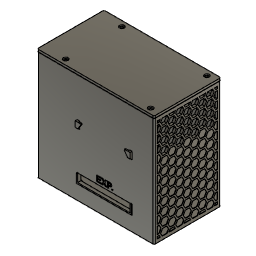
book8088_isa_exp_encloser_typeA (Autodesk Fusion 360 design; units mm, degrees)
Autodesk Fusion 360 part; units mm, degrees
(part 1 of 3)
sketch "스케치1" plane through (0, 0, 0) normal (0, 0, 1) x (1, 0, 0)
  line L0 (0, 75.3) -> (90.25, 75.3)
  line L1 (90.25, 75.3) -> (90.25, 0) construction
  line L2 (90.25, 0) -> (0, 0)
  line L3 (0, 0) -> (0, 75.3) construction
  line L4 (1.75, 0) -> (22.5, 0)
  line L5 (0, 1.75) -> (0, 22.5)
  line L6 (4.35, 70.95) -> (4.35, 4.35) construction
  line L7 (85.9, 70.95) -> (85.9, 4.35) construction
  line L8 (4.35, 70.95) -> (85.9, 70.95) construction
  line L9 (4.35, 4.35) -> (85.9, 4.35) construction
  circle A0 centre (4.35, 70.95) radius 1.55
  circle A1 centre (4.35, 70.95) radius 5
  circle A2 centre (85.9, 70.95) radius 1.55
  circle A3 centre (85.9, 70.95) radius 5
  circle A4 centre (85.9, 4.35) radius 1.55
  circle A5 centre (85.9, 4.35) radius 5
  circle A6 centre (4.35, 4.35) radius 1.55
  circle A7 centre (4.35, 4.35) radius 5
  line L10 (-37, 78.3) -> (105.25, 78.3)
  line L11 (105.25, 78.3) -> (105.25, -3)
  line L12 (105.25, -3) -> (-37, -3)
  line L13 (-37, -3) -> (-37, 78.3)
  line L14 (102.25, 75.3) -> (102.25, 0)
  line L15 (90.25, 75.3) -> (102.25, 75.3)
  line L16 (102.25, 0) -> (90.25, 0)
  line L17 (-34, 75.3) -> (-34, 0)
  line L18 (-34, 75.3) -> (0, 75.3)
  line L19 (-34, 0) -> (0, 0)
  line L20 (-22.25, 75.3) -> (-22.25, 0)
  line L21 (-25.75, 75.3) -> (-25.75, 0)
  line L22 (-22.25, 67.225) -> (-25.75, 67.225)
  line L23 (-25.75, 54.875) -> (-22.25, 54.875)
  line L24 (-25.75, 46.825) -> (-22.25, 46.825)
  line L25 (-25.75, 34.475) -> (-22.25, 34.475)
  line L26 (-25.75, 26.425) -> (-22.25, 26.425)
  line L27 (-22.25, 14.075) -> (-25.75, 14.075)
  line L28 (-22.25, 54.875) -> (-19.75, 54.875)
  line L29 (-19.75, 54.875) -> (-19.75, 67.225)
  line L30 (-19.75, 67.225) -> (-22.25, 67.225)
  line L31 (-22.25, 46.825) -> (-19.75, 46.825)
  line L32 (-19.75, 46.825) -> (-19.75, 34.475)
  line L33 (-19.75, 34.475) -> (-22.25, 34.475)
  line L34 (-22.25, 26.425) -> (-19.75, 26.425)
  line L35 (-19.75, 26.425) -> (-19.75, 14.075)
  line L36 (-19.75, 14.075) -> (-22.25, 14.075)
  circle A8 centre (-27.33, 69.325) radius 1.5
  line L37 (-34, 67.825) -> (-25.75, 67.825) construction
  line L38 (-25.83, 75.3) -> (-25.83, 0) construction
  line L39 (-33.7, 47.425) -> (-26.25, 47.425) construction
  circle A9 centre (-27.33, 48.925) radius 1.5
  circle A10 centre (-27.33, 28.525) radius 1.5
  line L40 (-33.7, 27.025) -> (-26.25, 27.025) construction
  line L41 (2.65, 59.35) -> (87.9, 59.35) construction
  line L42 (87.9, 59.35) -> (87.9, 50.4) construction
  line L43 (87.9, 50.4) -> (2.65, 50.4) construction
  line L44 (2.65, 50.4) -> (2.65, 59.35) construction
  line L45 (87.9, 30) -> (2.65, 30) construction
  line L46 (2.65, 38.95) -> (87.9, 38.95) construction
  line L47 (2.65, 30) -> (2.65, 38.95) construction
  line L48 (87.9, 38.95) -> (87.9, 30) construction
  line L49 (87.9, 9.6) -> (2.65, 9.6) construction
  line L50 (2.65, 18.55) -> (87.9, 18.55) construction
  line L51 (2.65, 9.6) -> (2.65, 18.55) construction
  line L52 (87.9, 18.55) -> (87.9, 9.6) construction
  line L53 (2.65, 54.875) -> (87.9, 54.875) construction
  line L54 (2.65, 34.475) -> (87.9, 34.475) construction
  line L55 (2.65, 14.075) -> (87.9, 14.075) construction
  line L56 (96.25, 59.35) -> (102.25, 59.35)
  line L57 (96.25, 50.4) -> (102.25, 50.4)
  line L58 (96.25, 59.35) -> (96.25, 56.375)
  line L59 (96.25, 56.375) -> (99.75, 56.375)
  line L60 (99.75, 56.375) -> (99.75, 53.375)
  line L61 (99.75, 53.375) -> (96.25, 53.375)
  line L62 (96.25, 53.375) -> (96.25, 50.4)
  line L63 (96.25, 38.95) -> (102.25, 38.95)
  line L64 (96.25, 38.95) -> (96.25, 35.975)
  line L65 (96.25, 35.975) -> (99.75, 35.975)
  line L66 (99.75, 35.975) -> (99.75, 32.975)
  line L67 (99.75, 32.975) -> (96.25, 32.975)
  line L68 (96.25, 32.975) -> (96.25, 30)
  line L69 (96.25, 30) -> (102.25, 30)
  line L70 (96.25, 18.55) -> (102.25, 18.55)
  line L71 (96.25, 18.55) -> (96.25, 15.575)
  line L72 (96.25, 15.575) -> (99.75, 15.575)
  line L73 (99.75, 15.575) -> (99.75, 12.575)
  line L74 (99.75, 12.575) -> (96.25, 12.575)
  line L75 (96.25, 12.575) -> (96.25, 9.6)
  line L76 (96.25, 9.6) -> (102.25, 9.6)
  line L77 (11.625, 0) -> (11.625, -3) construction
  line L78 (78.625, 0) -> (78.625, -3) construction
  line L79 (45.125, 0) -> (45.125, -3) construction
  line L80 (10.25, 78.3) -> (10.25, 75.3) construction
  line L81 (17.95, 78.3) -> (17.95, 75.3) construction
  line L82 (-37, 75.3) -> (-34, 75.3)
  line L83 (-37, 0) -> (-34, 0)
  line L84 (-22.25, 69.225) -> (-17.75, 69.225)
  line L85 (-17.75, 69.225) -> (-17.75, 52.875)
  line L86 (-17.75, 52.875) -> (-22.25, 52.875)
  line L87 (-17.75, 61.05) -> (-19.75, 61.05) construction
  line L88 (-22.25, 48.825) -> (-17.75, 48.825)
  line L89 (-17.75, 48.825) -> (-17.75, 32.475)
  line L90 (-17.75, 40.65) -> (-19.75, 40.65) construction
  line L91 (-17.75, 32.475) -> (-22.25, 32.475)
  line L92 (-22.25, 28.425) -> (-17.75, 28.425)
  line L93 (-17.75, 28.425) -> (-17.75, 12.075)
  line L94 (-17.75, 20.25) -> (-19.75, 20.25) construction
  line L95 (-17.75, 12.075) -> (-22.25, 12.075)
  line L96 (-37, 9.6) -> (-22.25, 9.6)
  line L97 (91.25, 0) -> (91.25, 7)
  line L98 (91.25, 7) -> (98.25, 7)
  line L99 (98.25, 7) -> (98.25, 0)
  circle A11 centre (94.75, 3.5) radius 3.5 construction
  circle A12 centre (94.75, 3.5) radius 1.5
  line L100 (91.25, 75.3) -> (91.25, 68.3)
  line L101 (91.25, 68.3) -> (98.25, 68.3)
  line L102 (98.25, 68.3) -> (98.25, 75.3)
  circle A13 centre (94.75, 71.8) radius 3.5 construction
  circle A14 centre (94.75, 71.8) radius 1.5
  line L103 (-12.25, 7) -> (-12.25, 0)
  line L104 (-12.25, 7) -> (-5.25, 7)
  line L105 (-5.25, 7) -> (-5.25, 0)
  line L106 (-12.25, 75.3) -> (-12.25, 68.3)
  line L107 (-12.25, 68.3) -> (-5.25, 68.3)
  line L108 (-5.25, 68.3) -> (-5.25, 75.3)
  circle A15 centre (-8.75, 71.8) radius 3.5 construction
  circle A16 centre (-8.75, 3.5) radius 3.5 construction
  circle A17 centre (-8.75, 3.5) radius 1.5
  circle A18 centre (-8.75, 71.8) radius 1.5
  dimension "d1" = 90.25
  dimension "d2" = 75.3
  dimension "d3" = 4.35
  dimension "d4" = 4.35
  dimension "d5" = 4.35
  dimension "d6" = 4.35
  dimension "d8" = 81.55
  dimension "d9" = 3.1
  dimension "d10" = 10
  dimension "d11" = 3
  dimension "d12" = 3
  dimension "d13" = 37
  dimension "d14" = 15
  dimension "d15" = 3
  dimension "d16" = 3
  dimension "d17" = 22.25
  dimension "d18" = 3.5
  dimension "d21" = 12.35
  dimension "d24" = 8.05
  dimension "d25" = 8.05
  dimension "d26" = 2.5
  dimension "d27" = 3
  dimension "d28" = 0.6
  dimension "d33" = 0.6
  dimension "d34" = 0.6
  dimension "d36" = 8.95
  dimension "d38" = 85.25
  dimension "d43" = 1.7
  dimension "d44" = 9.6
  dimension "d46" = 3
  dimension "d47" = 6
  dimension "d48" = 3.5
  dimension "d55" = 67
  dimension "d56" = 7.7
  dimension "d57" = 5.9
  dimension "d94" = 2
  dimension "d95" = 2
  dimension "d104" = 3.58
  dimension "d146" = 7
  dimension "d147" = 7
  dimension "d149" = 3
  dimension "d150" = 4
  dimension "d151" = 10
  constraint horizontal L0
  constraint vertical L1
  constraint horizontal L2
  constraint vertical L3
  constraint collinear L2 L4
  constraint collinear L3 L5
  constraint perpendicular L2 L6
  constraint horizontal L8
  constraint horizontal L9
  constraint equal L8 L9
  constraint equal L6 L7
  constraint perpendicular L7 L8
  constraint coincident L6 L8.start
  constraint coincident L8 L6.start
  constraint concentric A0 A1
  constraint equal A0 A2
  constraint equal A0 A6
  constraint equal A0 A4
  constraint equal A1 A3
  constraint equal A1 A7
  constraint equal A1 A5
  constraint coincident L7 L8.end
  constraint coincident L8 L7.start
  constraint coincident L7 L9.end
  constraint coincident L9 L7.end
  constraint coincident L9 L6.end
  constraint coincident L6 L9.start
  constraint concentric A2 A3
  constraint concentric A4 A5
  constraint concentric A6 A7
  constraint coincident L7.end L9.end
  constraint coincident L7.start L8.end
  constraint coincident L6.start L8.start
  constraint coincident L6.end L9.start
  constraint horizontal L10
  constraint perpendicular L10 L11
  constraint perpendicular L11 L12
  constraint perpendicular L10 L13
  constraint coincident L10.start L13.end
  constraint parallel L1 L14
  constraint perpendicular L1 L15
  constraint collinear L0 L15
  constraint coincident L0.end L1.start
  constraint coincident L14.start L15.end
  constraint horizontal L16
  constraint collinear L2 L16
  constraint coincident L1.end L2.start
  constraint coincident L14.end L16.start
  constraint perpendicular L12 L17
  constraint coincident L2.end L3.start
  constraint collinear L0 L18
  constraint collinear L2 L19
  constraint parallel L17 L20
  constraint coincident L18 L20.start
  constraint coincident L19 L20.end
  constraint parallel L20 L21
  constraint coincident L18 L21.start
  constraint coincident L19 L21.end
  constraint coincident L20 L22.start
  constraint coincident L21 L22.end
  constraint perpendicular L21 L22
  constraint coincident L21 L23.start
  constraint coincident L20 L23.end
  constraint perpendicular L20 L23
  constraint coincident L21 L24.start
  constraint coincident L20 L24.end
  constraint perpendicular L20 L24
  constraint coincident L21 L25.start
  constraint coincident L20 L25.end
  constraint perpendicular L20 L25
  constraint coincident L21 L26.start
  constraint coincident L20 L26.end
  constraint perpendicular L20 L26
  constraint coincident L20 L27.start
  constraint coincident L21 L27.end
  constraint perpendicular L21 L27
  constraint perpendicular L20 L28
  constraint perpendicular L23 L29
  constraint perpendicular L24 L32
  constraint perpendicular L26 L35
  constraint collinear L26 L34
  constraint collinear L27 L36
  constraint collinear L25 L33
  constraint collinear L24 L31
  constraint collinear L22 L30
  constraint equal L30 L31
  constraint equal L30 L34
  constraint horizontal L37
  constraint tangent A8 L37
  constraint coincident L21 L37.end
  constraint coincident L17 L37.start
  constraint vertical L38
  constraint tangent A8 L38
  constraint coincident L18 L38.start
  constraint coincident L19 L38.end
  constraint horizontal L39
  constraint tangent L39 A9
  constraint horizontal L40
  constraint tangent A10 L40
  constraint equal A8 A9
  constraint equal A8 A10
  constraint horizontal L41
  constraint vertical L42
  constraint horizontal L43
  constraint vertical L44
  constraint equal L29 L32
  constraint equal L29 L35
  constraint horizontal L46
  constraint vertical L48
  constraint horizontal L45
  constraint vertical L47
  constraint horizontal L50
  constraint vertical L52
  constraint horizontal L49
  constraint vertical L51
  constraint equal L41 L45
  constraint equal L41 L50
  constraint equal L42 L48
  constraint equal L42 L52
  constraint collinear L42 L48
  constraint collinear L42 L52
  constraint parallel L0 L53
  constraint symmetric L41 L43 L53
  constraint coincident L44 L53.start
  constraint coincident L42 L53.end
  constraint symmetric L45 L46 L54
  constraint symmetric L49 L50 L55
  constraint coincident L47 L54.start
  constraint coincident L48 L54.end
  constraint coincident L52 L55.end
  constraint coincident L51 L55.start
  constraint collinear L36 L55
  constraint collinear L33 L54
  constraint collinear L28 L53
  constraint perpendicular L1 L56
  constraint perpendicular L1 L57
  constraint equal L56 L57
  constraint collinear L41 L56
  constraint collinear L43 L57
  constraint coincident L14 L56.end
  constraint coincident L14 L57.end
  constraint perpendicular L56 L58
  constraint perpendicular L1 L59
  constraint perpendicular L59 L60
  constraint perpendicular L1 L61
  constraint perpendicular L57 L62
  constraint symmetric L53 L59 L61
  constraint equal L63 L69
  constraint perpendicular L63 L64
  constraint perpendicular L65 L66
  constraint perpendicular L68 L69
  constraint equal L70 L76
  constraint perpendicular L70 L71
  constraint perpendicular L72 L73
  constraint perpendicular L75 L76
  constraint coincident L14 L63.end
  constraint coincident L14 L69.end
  constraint coincident L14 L70.end
  constraint coincident L14 L76.end
  constraint collinear L46 L63
  constraint collinear L45 L69
  constraint collinear L50 L70
  constraint collinear L49 L76
  constraint symmetric L55 L72 L74
  constraint symmetric L54 L65 L67
  constraint perpendicular L66 L67
  constraint perpendicular L73 L74
  constraint equal L56 L63
  constraint equal L59 L65
  constraint equal L60 L66
  constraint equal L56 L70
  constraint equal L59 L72
  constraint equal L60 L73
  constraint coincident L2 L77.start
  constraint coincident L12 L77.end
  constraint perpendicular L12 L77
  constraint coincident L2 L78.start
  constraint coincident L12 L78.end
  constraint perpendicular L12 L78
  constraint coincident L2 L79.start
  constraint coincident L12 L79.end
  constraint perpendicular L12 L79
  constraint symmetric L77 L78 L79
  constraint symmetric L6 L7 L79
  constraint coincident L10 L80.start
  constraint coincident L0 L80.end
  constraint perpendicular L0 L80
  constraint coincident L10 L81.start
  constraint coincident L0 L81.end
  constraint perpendicular L0 L81
  constraint perpendicular L13 L82
  constraint collinear L18 L82
  constraint coincident L17.start L18.start
  constraint coincident L13 L82.start
  constraint horizontal L83
  constraint collinear L19 L83
  constraint coincident L17.end L19.start
  constraint coincident L13 L83.start
  constraint tangent L38 A9
  constraint tangent L38 A10
  constraint coincident L20 L84.start
  constraint perpendicular L20 L84
  constraint perpendicular L10 L85
  constraint coincident L20 L86.end
  constraint perpendicular L20 L86
  constraint coincident L85 L87.start
  constraint coincident L29 L87.end
  constraint perpendicular L29 L87
  constraint symmetric L28 L30 L87
  constraint symmetric L84 L86 L87
  constraint coincident L90.start L89
  constraint symmetric L88 L90 L91
  constraint coincident L94.start L93
  constraint symmetric L92 L94 L95
  constraint coincident L20 L88.start
  constraint coincident L32 L90.end
  constraint coincident L20 L91.end
  constraint coincident L20 L92.start
  constraint coincident L35 L94.end
  constraint coincident L20 L95.end
  constraint symmetric L34 L36 L94
  constraint symmetric L31 L33 L90
  constraint perpendicular L93 L95
  constraint perpendicular L92 L93
  constraint perpendicular L89 L91
  constraint perpendicular L88 L89
  constraint equal L87 L90
  constraint equal L87 L94
  constraint equal L85 L89
  constraint equal L85 L93
  constraint perpendicular L17 L96
  constraint collinear L49 L96
  constraint coincident L20 L96.end
  constraint coincident L13 L96.start
  constraint perpendicular L9 L97
  constraint perpendicular L97 L98
  constraint perpendicular L98 L99
  constraint coincident L2 L99.end
  constraint coincident L2 L97.start
  constraint tangent L98 A11
  constraint tangent L99 A11
  constraint tangent L97 A11
  constraint concentric A11 A12
  constraint perpendicular L8 L100
  constraint perpendicular L100 L101
  constraint perpendicular L8 L102
  constraint coincident L0 L100.start
  constraint coincident L0 L102.end
  constraint equal L98 L101
  constraint equal L99 L102
  constraint tangent L102 A13
  constraint tangent L101 A13
  constraint tangent L100 A13
  constraint concentric A13 A14
  constraint equal A12 A14
  constraint collinear L97 L100
  constraint coincident L19 L103.end
  constraint perpendicular L19 L103
  constraint perpendicular L20 L104
  constraint coincident L19 L105.end
  constraint perpendicular L19 L105
  constraint coincident L18 L106.start
  constraint perpendicular L18 L106
  constraint perpendicular L106 L107
  constraint coincident L18 L108.end
  constraint perpendicular L18 L108
  constraint equal L98 L104
  constraint equal L98 L107
  constraint equal L99 L105
  constraint equal L99 L108
  constraint collinear L103 L106
  constraint tangent L105 A16
  constraint tangent L104 A16
  constraint tangent L103 A16
  constraint tangent L108 A15
  constraint tangent L107 A15
  constraint tangent L106 A15
  constraint equal A12 A18
  constraint equal A12 A17
  constraint concentric A16 A17
  constraint concentric A15 A18
  measures "d1" distance of L1.end L2.end
  measures "d2" distance of L0.end L1.end
  measures "d3" distance of L2 L9
  measures "d4" distance of L1 L7
  measures "d5" distance of L0 L8
  measures "d6" distance of L3 L6
  measures "d8" distance of L6 L7
  measures "d9" diameter of A0
  measures "d10" diameter of A1
  measures "d11" distance of L0 L10
  measures "d12" distance of L2 L12
  measures "d13" distance of L3 L13
  measures "d14" distance of L1 L11
  measures "d15" distance of L11 L14
  measures "d16" distance of L13 L17
  measures "d17" distance of L3 L20
  measures "d18" distance of L20 L21
  measures "d21" distance of L22 L23
  measures "d24" distance of L23 L24
  measures "d25" distance of L25 L26
  measures "d26" distance of L22.start L29.end
  measures "d27" diameter of A8
  measures "d28" distance of L22 L37
  measures "d33" distance of L24 L39
  measures "d34" distance of L26 L40
  measures "d36" distance of L41.end L42.end
  measures "d38" distance of L41.start L41.end
  measures "d43" distance of L6 L44
  measures "d44" distance of L2 L49
  measures "d46" distance of L59.end L60.end
  measures "d47" distance of L56.start L56.end
  measures "d48" distance of L58.end L59.end
  measures "d55" distance of L77 L78
  measures "d56" distance of L80 L81
  measures "d57" distance of L6 L80
  measures "d94" distance of L87.start L87.end
  measures "d95" distance of L30 L84
  measures "d104" distance of L20 L38
  measures "d146" distance of L98.end L99.end
  measures "d147" distance of L97.end L98.end
  measures "d149" diameter of A12
  measures "d150" distance of L14 L102
  measures "d151" distance of L20 L103
extrude "돌출1" add sketch "스케치1" along normal blind 2.5 contours L0 L2 L4 A1 A3 A5 A7 L10 L11 L12 L13 L14 L15 L16 L18 L19 L82 L83 | L0 L2 L4 A1 A3 A5 A7 L14 L15 L16 L18 L19 L20 L56 L57 L58 L59 L60 L61 L62 L63 L64 L65 L66 L67 L68 L69 L70 L71 L72 L73 L74 L75 L76 L84 L85 L86 L88 L89 L91 L92 L93 L95 L97 L98 L99 L100 L101 L102 L103 L104 L105 L106 L107 L108 | L0 A1 | L0 A1 | L18 L106 L107 L108 | L0 A3 | L0 A3 | L18 L20 L21 L22 | L17 L18 L21 L96 | L20 L28 L29 L30 L84 L85 L86 | L13 L17 L82 L96 | L20 L21 L22 L23 | L20 L28 L29 L30 | L15 L100 L101 L102 | L17 L19 L21 L96 | L13 L17 L83 L96 | L20 L21 L23 L24 | L19 L20 L21 L96 | L20 L21 L27 L96 | L20 L21 L24 L25 | L20 L21 L26 L27 | L20 L21 L25 L26 | L20 L31 L32 L33 | L20 L31 L32 L33 L88 L89 L91 | L14 L56 L57 L58 L59 L60 L61 L62 | L20 L34 L35 L36 L92 L93 L95 | L20 L34 L35 L36 | L19 L103 L104 L105 | L14 L63 L64 L65 L66 L67 L68 L69 | L14 L70 L71 L72 L73 L74 L75 L76 | L2 L4 L5 A7 | L2 L4 A7 | L5 A7 | L16 L97 L98 L99 | L2 A5 | L2 A5 | A0 | A2 | A4 | A6 | A8 | A9 | A10 | A12 | A14 | A17 | A18 makes body 1
extrude "돌출2" cut sketch "스케치1" along normal through all and the other way blind 1.5 from surface at 2.5 contours L20 L28 L29 L30 | L20 L31 L32 L33 | L20 L34 L35 L36 bodies 1
extrude "돌출13" add sketch "스케치1" along normal blind 6.5 contours L20 L28 L29 L30 L84 L85 L86 | L20 L31 L32 L33 L88 L89 L91 | L20 L34 L35 L36 L92 L93 L95 bodies 1
extrude "돌출3" add sketch "스케치1" along normal blind 11.5 contours L0 A1 | L0 A1 | L0 A3 | L0 A3 | L2 L4 L5 A7 | L2 L4 A7 | L5 A7 | L2 A5 | L2 A5 bodies 1
extrude "돌출4" add sketch "스케치1" along normal blind 132.5 contours L0 L2 L4 A1 A3 A5 A7 L10 L11 L12 L13 L14 L15 L16 L18 L19 L82 L83 | L0 A1 | L0 A3 | L2 L4 A7 | L2 A5 picked at (4.2274, 75.722) picked at (86.0226, 75.5121) picked at (86.5, -0.1049) bodies 1
extrude "돌출5" add sketch "스케치1" along normal blind 118.5 contours L18 L20 L21 L22 | L20 L21 L23 L24 | L19 L20 L21 L96 | L20 L21 L27 L96 | L20 L21 L25 L26 bodies 1
extrude "돌출12" add sketch "스케치1" along normal blind 21.5 contours L20 L21 L22 L23 | L20 L21 L24 L25 | L20 L21 L26 L27 bodies 1
extrude "돌출6" add sketch "스케치1" along normal blind 3 from surface at 118.5 contours L18 L20 L21 L22 | L17 L18 L21 L96 | L20 L21 L22 L23 | L17 L19 L21 L96 | L20 L21 L23 L24 | L19 L20 L21 L96 | L20 L21 L27 L96 | L20 L21 L24 L25 | L20 L21 L26 L27 | L20 L21 L25 L26 bodies 1
extrude "돌출17" add sketch "스케치1" along normal blind 132.5 contours L17 L19 L21 L96 | L13 L17 L83 L96 | L19 L20 L21 L96 bodies 1
extrude "돌출7" add sketch "스케치1" along normal blind 50 from surface at 31.5 contours L14 L56 L57 L58 L59 L60 L61 L62 | L14 L63 L64 L65 L66 L67 L68 L69 | L14 L70 L71 L72 L73 L74 L75 L76 bodies 1
chamfer "모따기9" distance 6 angle 45 3 edges at (102.25, 14.075, 81.5) (102.25, 34.475, 81.5) (102.25, 54.875, 81.5) on bodies 1
chamfer "모따기10" distance 6 angle 45 3 edges at (102.25, 54.875, 31.5) (102.25, 34.475, 31.5) (102.25, 14.075, 31.5) on bodies 1
extrude "돌출26" add sketch "스케치1" against normal blind 10 from surface at 132.5 contours L18 L106 L107 L108 | L15 L100 L101 L102 | L19 L103 L104 L105 | L16 L97 L98 L99 | A12 | A14 | A17 | A18 bodies 1
chamfer "모따기5" distance 7 angle 45 2 edges at (94.75, 75.3, 122.5) (-8.75, 75.3, 122.5) on bodies 1
chamfer "모따기6" distance 7 angle 45 2 edges at (94.75, 0, 122.5) (-8.75, 0, 122.5) on bodies 1
extrude "돌출27" cut sketch "스케치1" against normal blind 9 from surface at 132.5 contours A12 | A14 | A17 | A18 bodies 1
sketch "스케치8" plane through (0, 0, 0) normal (0, 0, -1) x (1, 0, 0)
  line L0 (-37, 3) -> (-37, -78.3)
  line L1 (-37, -78.3) -> (105.25, -78.3)
  line L2 (105.25, -78.3) -> (105.25, 3)
  line L3 (105.25, 3) -> (-37, 3)
  circle A0 centre (-22, -12) radius 10
  circle A1 centre (90.25, -12) radius 10
  circle A2 centre (90.25, -63.3) radius 10
  circle A3 centre (-22, -63.3) radius 10
  line L4 (-32, 3) -> (-32, -78.3) construction
  line L5 (100.25, 3) -> (100.25, -78.3) construction
  line L6 (-37, -2) -> (105.25, -2) construction
  line L7 (-37, -73.3) -> (105.25, -73.3) construction
  line L8 (-37, 3) -> (-37, -78.3)
  line L9 (105.25, -78.3) -> (105.25, 3)
  line L10 (105.25, 3) -> (-37, 3)
  line L11 (-37, -78.3) -> (105.25, -78.3)
  line L12 (-22, -2) -> (-22, -22)
  line L13 (-32, -12) -> (-12, -12)
  line L14 (-32, -63.3) -> (-12, -63.3)
  line L15 (-22, -53.3) -> (-22, -73.3)
  line L16 (90.25, -53.3) -> (90.25, -73.3)
  line L17 (80.25, -63.3) -> (100.25, -63.3)
  line L18 (80.25, -12) -> (100.25, -12)
  line L19 (90.25, -22) -> (90.25, -2)
  circle A4 centre (-22, -63.3) radius 8
  circle A5 centre (-22, -12) radius 8
  circle A6 centre (90.25, -12) radius 8
  circle A7 centre (90.25, -63.3) radius 8
  line L20 (-32, -13) -> (-12, -13)
  line L21 (-32, -11) -> (-12, -11)
  line L22 (-23, -2) -> (-23, -22)
  line L23 (-21, -2) -> (-21, -22)
  line L24 (-32, -64.3) -> (-12, -64.3)
  line L25 (-32, -62.3) -> (-12, -62.3)
  line L26 (-23, -53.3) -> (-23, -73.3)
  line L27 (-21, -53.3) -> (-21, -73.3)
  line L28 (80.25, -64.3) -> (100.25, -64.3)
  line L29 (80.25, -62.3) -> (100.25, -62.3)
  line L30 (89.25, -53.3) -> (89.25, -73.3)
  line L31 (91.25, -53.3) -> (91.25, -73.3)
  line L32 (80.25, -13) -> (100.25, -13)
  line L33 (80.25, -11) -> (100.25, -11)
  line L34 (91.25, -22) -> (91.25, -2)
  line L35 (89.25, -22) -> (89.25, -2)
  dimension "d218" = 5
  dimension "d219" = 5
  dimension "d220" = 5
  dimension "d221" = 5
  dimension "d222" = 20
  dimension "d223" = -2
  dimension "d224" = -2
  dimension "d225" = -2
  dimension "d226" = -2
  dimension "d227" = 1
  dimension "d228" = -1
  dimension "d229" = 1
  dimension "d230" = -1
  dimension "d231" = 1
  dimension "d232" = -1
  dimension "d233" = 1
  dimension "d234" = -1
  dimension "d235" = 1
  dimension "d236" = -1
  dimension "d237" = 1
  dimension "d238" = -1
  dimension "d239" = 1
  dimension "d240" = -1
  dimension "d241" = 1
  dimension "d242" = -1
  constraint equal A0 A1
  constraint equal A0 A2
  constraint equal A0 A3
  constraint perpendicular L3 L4
  constraint perpendicular L2 L6
  constraint horizontal L7
  constraint tangent A1 L6
  constraint tangent A1 L5
  constraint tangent A2 L5
  constraint tangent A2 L7
  constraint tangent A3 L7
  constraint tangent A3 L4
  constraint tangent A0 L4
  constraint tangent A0 L6
  constraint perpendicular L5 L6
  constraint equal L4 L5
  constraint equal L6 L7
  constraint coincident L5.start L10
  constraint coincident L5.end L11
  constraint coincident L7.end L9
  constraint coincident L6.end L9
  constraint coincident L4.start L10
  constraint coincident L7.start L8
  constraint parallel L4 L12
  constraint horizontal L14
  constraint vertical L15
  constraint vertical L16
  constraint perpendicular L18 L19
  constraint perpendicular L16 L17
  constraint perpendicular L12 L13
  constraint parallel L6 L18
  constraint coincident A1.centre L18
  constraint coincident A1.centre L19
  constraint coincident A1 L19.start
  constraint coincident A1 L19.end
  constraint coincident A1 L18.end
  constraint coincident A1 L18.start
  constraint coincident A2 L16.start
  constraint coincident A2 L16.end
  constraint coincident A2.centre L16
  constraint coincident A2.centre L17
  constraint coincident A2 L17.end
  constraint coincident A2 L17.start
  constraint coincident A3.centre L15
  constraint coincident A3.centre L14
  constraint coincident A3 L14.end
  constraint coincident A3 L14.start
  constraint coincident A3 L15.start
  constraint coincident A3 L15.end
  constraint coincident A0.centre L13
  constraint coincident A0.centre L12
  constraint coincident A0 L12.end
  constraint coincident A0 L12.start
  constraint coincident A0 L13.end
  constraint coincident A0 L13.start
  measures "d218" distance of L4 L8
  measures "d219" distance of L5 L9
  measures "d220" distance of L6 L10
  measures "d221" distance of L7 L11
  measures "d222" diameter of A0
extrude "돌출41" cut sketch "스케치8" against normal blind 0.4 contours L13 A5 L20 L23 | L13 A5 L21 L23 | L12 A5 L20 L23 | L12 A5 L20 L22 | L19 A6 L32 L34 | L19 A6 L32 L35 | L18 A6 L32 L35 | L18 A6 L33 L35 | L16 A7 L29 L31 | L16 A7 L29 L30 | L17 A7 L28 L30 | L17 A7 L29 L30 | L14 A4 L24 L27 | L14 A4 L25 L27 | L15 A4 L25 L27 | L15 A4 L25 L26 bodies 1
sketch "스케치7" plane through (-25.75, 0, 0) normal (-1, 0, 0) x (0, -1, 0)
  line L0 (-9.6, 2.5) -> (-9.6, 118.5)
  line L1 (-9.6, 118.5) -> (-14.075, 118.5)
  line L2 (-14.075, 118.5) -> (-14.075, 21.5)
  line L3 (-14.075, 21.5) -> (-26.425, 21.5)
  line L4 (-26.425, 21.5) -> (-26.425, 118.5)
  line L5 (-26.425, 118.5) -> (-34.475, 118.5)
  line L6 (-34.475, 118.5) -> (-34.475, 21.5)
  line L7 (-34.475, 21.5) -> (-46.825, 21.5)
  line L8 (-46.825, 21.5) -> (-46.825, 118.5)
  line L9 (-46.825, 118.5) -> (-54.875, 118.5)
  line L10 (-54.875, 118.5) -> (-54.875, 21.5)
  line L11 (-54.875, 21.5) -> (-67.225, 21.5)
  line L12 (-67.225, 21.5) -> (-67.225, 118.5)
  line L13 (-67.225, 118.5) -> (-75.3, 118.5)
  line L14 (-75.3, 118.5) -> (-75.3, 2.5)
  line L15 (-75.3, 2.5) -> (-9.6, 2.5)
  line L16 (-26.425, 7.5) -> (-14.075, 7.5) construction
  line L17 (-14.075, 7.5) -> (-14.075, 17.5) construction
  line L18 (-14.075, 17.5) -> (-26.425, 17.5) construction
  line L19 (-26.425, 17.5) -> (-26.425, 7.5) construction
  line L20 (-46.825, 7.5) -> (-34.475, 7.5) construction
  line L21 (-34.475, 7.5) -> (-34.475, 17.5) construction
  line L22 (-34.475, 17.5) -> (-46.825, 17.5) construction
  line L23 (-46.825, 17.5) -> (-46.825, 7.5) construction
  line L24 (-67.225, 7.5) -> (-54.875, 7.5) construction
  line L25 (-54.875, 7.5) -> (-54.875, 17.5) construction
  line L26 (-54.875, 17.5) -> (-67.225, 17.5) construction
  line L27 (-67.225, 17.5) -> (-67.225, 7.5) construction
  dimension "d205" = 7
  dimension "d206" = 4
  dimension "d207" = 10
  dimension "d208" = 7
  dimension "d210" = 7
  dimension "d212" = 4
  dimension "d213" = 4
  text T0 "1" font "Arial" height 7 bold align centre middle in box 12.35 x 10 at (-26.425, 7.5) x (1, 0) y (0, 1) spacing 1 kerned
  text T1 "2" font "Arial" height 7 bold align centre middle in box 12.35 x 10 at (-46.825, 7.5) x (1, 0) y (0, 1) spacing 1 kerned
  text T2 "3" font "Arial" height 7 bold align centre middle in box 12.35 x 10 at (-67.225, 7.5) x (1, 0) y (0, 1) spacing 1 kerned
  constraint collinear L4 L19
  constraint collinear L2 L17
  constraint equal L18 L22
  constraint equal L18 L26
  constraint equal L19 L23
  constraint equal L19 L27
  constraint collinear L6 L21
  constraint collinear L10 L25
  measures "d206" distance of L3 L18
  measures "d212" distance of L7 L22
  measures "d213" distance of L11 L26
extrude "돌출39" cut sketch "스케치7" against normal blind 0.5 text T0 T1 T2 bodies 1
sketch "Exp_Cable" plane through (0, -3, 0) normal (0, -1, 0) x (1, 0, 0)
  line L0 (-37, 0) -> (105.25, 0)
  line L1 (105.25, 0) -> (105.25, 132.5)
  line L2 (105.25, 132.5) -> (-37, 132.5)
  line L3 (-37, 132.5) -> (-37, 0)
  line L4 (11.625, 132.5) -> (11.625, 0) construction
  line L5 (78.625, 132.5) -> (78.625, 0) construction
  line L6 (-37, 13.1) -> (105.25, 13.1) construction
  line L7 (105.25, 0) -> (-37, 0)
  line L8 (13.225, 28.1) -> (77.025, 28.1)
  line L9 (77.025, 28.1) -> (77.025, 19.9)
  line L10 (77.025, 19.9) -> (13.225, 19.9)
  line L11 (13.225, 19.9) -> (13.225, 28.1)
  line L12 (11.625, 85.1) -> (18.625, 85.1)
  line L13 (11.625, 78.1) -> (11.625, 85.1)
  line L14 (14.625, 85.1) -> (14.625, 78.1)
  line L15 (14.625, 83.9) -> (18.625, 83.9)
  line L16 (14.625, 78.1) -> (11.625, 78.1)
  line L17 (18.625, 83.9) -> (18.625, 85.1)
  line L18 (18.625, 83.9) -> (14.625, 78.1)
  line L19 (71.625, 85.1) -> (75.625, 85.1)
  line L20 (75.625, 85.1) -> (75.625, 83.9)
  line L21 (75.625, 83.9) -> (71.625, 83.9)
  line L22 (71.625, 83.9) -> (71.625, 85.1)
  line L23 (75.625, 85.1) -> (78.625, 85.1)
  line L24 (78.625, 85.1) -> (78.625, 78.1)
  line L25 (75.625, 78.1) -> (75.625, 83.9)
  line L26 (71.625, 83.9) -> (75.625, 78.1)
  line L27 (75.625, 78.1) -> (78.625, 78.1)
  line L28 (11.625, 30.1) -> (78.625, 30.1) construction
  line L29 (78.625, 30.1) -> (78.625, 40.1) construction
  line L30 (78.625, 40.1) -> (11.625, 40.1) construction
  line L31 (11.625, 40.1) -> (11.625, 30.1) construction
  line L32 (78.525, 18.4) -> (11.725, 18.4)
  line L33 (11.725, 18.4) -> (11.725, 29.6)
  line L34 (11.725, 29.6) -> (78.525, 29.6)
  line L35 (78.525, 29.6) -> (78.525, 18.4)
  line L36 (45.125, 28.1) -> (45.125, 19.9) construction
  line L37 (13.225, 28.1) -> (13.225, 29.6)
  line L38 (77.025, 28.1) -> (77.025, 29.6)
  point P0 (11.625, 0)
  point P1 (78.625, 0)
  dimension "d73" = 13.1
  dimension "d74" = 8.2
  dimension "d119" = 7
  dimension "d120" = 3
  dimension "d130" = 7
  dimension "d131" = 1.2
  dimension "d132" = 50
  dimension "d168" = 7
  dimension "d169" = 2
  dimension "d170" = 10
  dimension "d198" = -1.5
  dimension "d286" = 6.8
  dimension "d287" = 63.8
  text T0 "EXP." font "Arial" height 7 bold align centre middle in box 67 x 10 at (11.625, 30.1) x (1, 0) y (0, 1) spacing 1 kerned
  constraint perpendicular L0 L4
  constraint coincident P0 L4.end
  constraint coincident P1 L5.end
  constraint coincident L2 L5.start
  constraint coincident L2 L4.start
  constraint perpendicular L5 L6
  constraint coincident L1 L6.end
  constraint coincident L3 L6.start
  constraint horizontal L8
  constraint vertical L9
  constraint horizontal L10
  constraint vertical L11
  constraint horizontal L12
  constraint vertical L13
  constraint coincident L12 L14.start
  constraint collinear L4 L13
  constraint coincident L14 L15.start
  constraint coincident L15.end L17.start
  constraint perpendicular L4 L16
  constraint perpendicular L12 L17
  constraint coincident L14.end L16.start
  constraint horizontal L19
  constraint vertical L20
  constraint horizontal L21
  constraint vertical L22
  constraint coincident L5 L23.end
  constraint perpendicular L5 L23
  constraint coincident L5 L24.end
  constraint perpendicular L24 L27
  constraint perpendicular L21 L25
  constraint equal L15 L21
  constraint equal L16 L27
  constraint equal L13 L24
  constraint collinear L16 L27
  constraint collinear L15 L21
  constraint collinear L5 L29
  constraint collinear L4 L31
  constraint coincident L8 L36.start
  constraint coincident L10 L36.end
  constraint perpendicular L8 L36
  constraint symmetric L4 L5 L36
  constraint coincident L34 L37.end
  constraint perpendicular L34 L37
  constraint coincident L34 L38.end
  constraint perpendicular L34 L38
  measures "d73" distance of L6 L7
  measures "d74" distance of L8.end L9.end
  measures "d119" distance of L12.start L12.end
  measures "d120" distance of L4 L14
  measures "d130" distance of L12 L16
  measures "d131" distance of L12 L15
  measures "d132" distance of L8 L16
  measures "d169" distance of L8 L28
  measures "d170" distance of L28 L30
  measures "d286" distance of L6 L10
  measures "d287" distance of L9 L11
extrude "돌출8" cut sketch "Exp_Cable" against normal blind 10 contours L8 L9 L10 L11 bodies 1
extrude "돌출21" add sketch "Exp_Cable" along normal blind 2.5 contours L12 L13 L14 L16 | L20 L23 L24 L25 L27 bodies 1
chamfer "모따기4" distance 2 angle 45 2 edges at (77.125, -3, 78.1) (13.125, -3, 78.1) on bodies 1
extrude "돌출22" add sketch "Exp_Cable" along normal blind 1.5 from surface at 1 contours L12 L14 L15 L17 | L14 L15 L18 | L19 L20 L21 L22 | L21 L25 L26 bodies 1
extrude "돌출56" add sketch "Exp_Cable" along normal blind 1 contours L9 L10 L11 L32 L33 L34 L35 L37 L38 bodies 1
chamfer "모따기11" distance 1 angle 45 1 edges at (45.125, -3, 18.4) on bodies 1
extrude "돌출33" cut sketch "Exp_Cable" against normal blind 1 text T0 bodies 1
chamfer "모따기12" distance 1 angle 45 1 edges at (45.125, -3, 28.1) on bodies 1
sketch "스케치4" plane through (0, 78.3, 0) normal (0, 1, 0) x (-1, 0, 0)
  line L0 (-105.25, 0) -> (37, 0)
  line L1 (37, 0) -> (37, 132.5)
  line L2 (37, 132.5) -> (-105.25, 132.5)
  line L3 (-105.25, 132.5) -> (-105.25, 0)
  line L4 (-17.95, 132.5) -> (-17.95, 0) construction
  line L5 (-10.25, 132.5) -> (-10.25, 0) construction
  line L6 (-105.25, 13.1) -> (37, 13.1) construction
  line L7 (37, 0) -> (-105.25, 0)
  circle A0 centre (-14.1, 19.95) radius 3.85
  line L8 (-17.95, 16.1) -> (-10.25, 16.1) construction
  line L9 (-91, 13.1) -> (34, 13.1)
  line L10 (34, 13.1) -> (34, 11.6)
  line L11 (34, 11.6) -> (-91, 11.6)
  line L12 (-91, 11.6) -> (-91, 13.1)
  line L13 (-9.25, 14.95) -> (4.75, 14.95) construction
  line L14 (4.75, 14.95) -> (4.75, 24.95) construction
  line L15 (4.75, 24.95) -> (-9.25, 24.95) construction
  line L16 (-9.25, 24.95) -> (-9.25, 14.95) construction
  line L17 (-17.95, 19.95) -> (-10.25, 19.95) construction
  line L18 (-105.25, 90.5) -> (37, 90.5) construction
  line L19 (37, 90.5) -> (37, 102.5) construction
  line L20 (37, 102.5) -> (-105.25, 102.5) construction
  line L21 (-105.25, 102.5) -> (-105.25, 90.5) construction
  line L22 (-105.25, 78.5) -> (37, 78.5) construction
  line L23 (37, 78.5) -> (37, 90.5) construction
  line L24 (37, 90.5) -> (-105.25, 90.5) construction
  line L25 (-105.25, 90.5) -> (-105.25, 78.5) construction
  point P0 (-10.25, 0)
  point P1 (-17.95, 0)
  dimension "d78" = 13.1
  dimension "d82" = 3
  dimension "d177" = 1.5
  dimension "d178" = 3
  dimension "d180" = 3
  dimension "d183" = 4
  dimension "d184" = 1
  dimension "d185" = 14
  dimension "d187" = 10
  dimension "d190" = 8
  dimension "d191" = 9
  dimension "d193" = 12
  dimension "d194" = 12
  dimension "d309" = 14.25
  dimension "d311" = 30
  text T0 "DC 12V" font "Arial" height 4 bold align centre middle in box 14 x 10 at (-9.25, 14.95) x (1, 0) y (0, 1) spacing 1 kerned
  text T1 "Book8088 & Hand386" font "Arial" height 8 bold align centre middle in box 142.25 x 12 at (-105.25, 90.5) x (1, 0) y (0, 1) spacing 1 kerned
  text T2 "ISA BUS EXPANSION" font "Arial" height 9 bold align centre middle in box 142.25 x 12 at (-105.25, 78.5) x (1, 0) y (0, 1) spacing 1 kerned
  constraint vertical L4
  constraint vertical L5
  constraint coincident P0 L5.end
  constraint coincident P1 L4.end
  constraint coincident L2 L5.start
  constraint coincident L2 L4.start
  constraint horizontal L6
  constraint coincident L1 L6.end
  constraint coincident L3 L6.start
  constraint tangent L4 A0
  constraint tangent L5 A0
  constraint perpendicular L4 L8
  constraint coincident L5 L8.end
  constraint coincident L4 L8.start
  constraint tangent A0 L8
  constraint horizontal L9
  constraint vertical L10
  constraint horizontal L11
  constraint vertical L12
  constraint perpendicular L4 L17
  constraint coincident L4 L17.start
  constraint coincident L5 L17.end
  constraint coincident A0.centre L17
  constraint collinear L1 L19
  constraint collinear L3 L21
  constraint collinear L1 L23
  constraint collinear L3 L25
  constraint collinear L18 L24
  measures "d78" distance of L6 L7
  measures "d82" distance of L6 L8
  measures "d177" distance of L9 L11
  measures "d178" distance of L8 L9
  measures "d180" distance of L1 L10
  measures "d184" distance of L5 L16
  measures "d193" distance of L20 L24
  measures "d194" distance of L22 L24
  measures "d309" distance of L3 L12
  measures "d311" distance of L2 L20
extrude "돌출9" cut sketch "스케치4" against normal blind 10 contours A0 bodies 1
extrude "돌출34" cut sketch "스케치4" against normal blind 0.5 contours L9 L10 L11 L12 bodies 1
chamfer "모따기8" distance 0.5 angle 45 1 edges at (28.5, 77.8, 11.6) on bodies 1
extrude "돌출35" cut sketch "스케치4" against normal blind 0.5 text T0 bodies 1
extrude "돌출36" cut sketch "스케치4" against normal blind 0.5 text T2 T1 bodies 1
sketch "스케치6" plane through (0, 0, 132.5) normal (0, 0, 1) x (-1, 0, 0)
  line L0 (37, -75.3) -> (12.25, -75.3)
  line L1 (-102.25, -75.3) -> (-102.25, 0)
  line L2 (-102.25, 0) -> (-98.25, 0)
  line L3 (22.25, 0) -> (22.25, -9.6)
  line L4 (22.25, -9.6) -> (37, -9.6)
  line L5 (37, -9.6) -> (37, 3)
  line L6 (37, 3) -> (-105.25, 3)
  line L7 (-105.25, 3) -> (-105.25, -78.3)
  line L8 (37, -78.3) -> (37, -75.3)
  line L9 (37, -78.3) -> (-105.25, -78.3)
  line L10 (-105.25, -78.3) -> (-105.25, 3)
  line L11 (-105.25, 3) -> (37, 3)
  line L12 (37, 3) -> (37, -78.3)
  line L13 (-105.25, -78.3) -> (-105.25, 3)
  line L14 (37, 3) -> (37, -78.3)
  line L15 (-13.225, 3) -> (-77.025, 3)
  line L16 (-105.25, -78.3) -> (37, -78.3)
  line L17 (37, -75.3) -> (22.25, -75.3)
  line L18 (22.25, -9.6) -> (37, -9.6)
  line L19 (34, -75.3) -> (0, -75.3)
  line L20 (37, -9.6) -> (22.25, -9.6)
  line L21 (22.25, -75.3) -> (22.25, 0)
  line L22 (22.25, -75.3) -> (-102.25, -75.3)
  line L23 (-102.25, -75.3) -> (-102.25, 0)
  line L24 (-102.25, 0) -> (22.25, 0)
  line L25 (22.25, 0) -> (22.25, -75.3)
  line L26 (-100.75, -1.5) -> (20.75, -1.5)
  line L27 (20.75, -1.5) -> (20.75, -73.8) construction
  line L28 (20.75, -73.8) -> (-100.75, -73.8)
  line L29 (-100.75, -73.8) -> (-100.75, -1.5)
  line L30 (20.75, -73.8) -> (22.25, -73.8)
  line L31 (20.75, -1.5) -> (22.25, -1.5)
  circle A0 centre (8.75, -71.8) radius 1.5
  circle A1 centre (8.75, -3.5) radius 1.5
  circle A2 centre (-94.75, -71.8) radius 1.5
  circle A3 centre (-94.75, -3.5) radius 1.5
  line L32 (12.25, -75.3) -> (12.25, -68.3)
  line L33 (12.25, -68.3) -> (5.25, -68.3)
  line L34 (5.25, -68.3) -> (5.25, -75.3)
  line L35 (5.25, -75.3) -> (-91.25, -75.3)
  line L36 (-91.25, -75.3) -> (-91.25, -68.3)
  line L37 (-91.25, -68.3) -> (-98.25, -68.3)
  line L38 (-98.25, -68.3) -> (-98.25, -75.3)
  line L39 (-98.25, -75.3) -> (-102.25, -75.3)
  line L40 (-98.25, 0) -> (-98.25, -7)
  line L41 (-98.25, -7) -> (-91.25, -7)
  line L42 (-91.25, -7) -> (-91.25, 0)
  line L43 (-91.25, 0) -> (5.25, 0)
  line L44 (5.25, 0) -> (5.25, -7)
  line L45 (5.25, -7) -> (12.25, -7)
  line L46 (12.25, -7) -> (12.25, 0)
  line L47 (12.25, 0) -> (22.25, 0)
  circle A4 centre (8.75, -71.8) radius 2.925
  circle A5 centre (-94.75, -71.8) radius 2.925
  circle A6 centre (-94.75, -3.5) radius 2.925
  circle A7 centre (8.75, -3.5) radius 2.925
  line L48 (34, -75.3) -> (34, -9.6)
  line L49 (-105.25, -78.3) -> (37, -78.3)
  dimension "d139" = 1.5
  dimension "d162" = 5.85
  constraint horizontal L9
  constraint vertical L10
  constraint horizontal L11
  constraint vertical L12
  constraint collinear L10 L13
  constraint collinear L12 L14
  constraint collinear L11 L15
  constraint collinear L9 L16
  constraint parallel L9 L17
  constraint collinear L17 L19
  constraint collinear L18 L20
  constraint coincident L4.end L5.start
  constraint coincident L12 L0.start
  constraint horizontal L22
  constraint vertical L23
  constraint horizontal L24
  constraint vertical L25
  constraint collinear L2 L24
  constraint collinear L1 L23
  constraint collinear L0 L22
  constraint collinear L21 L25
  constraint coincident L25 L30.end
  constraint perpendicular L25 L30
  constraint perpendicular L21 L31
  constraint coincident L25 L31.end
  constraint equal A4 A5
  constraint equal A4 A7
  constraint equal A4 A6
  constraint concentric A0 A4
  constraint concentric A2 A5
  constraint concentric A3 A6
  constraint concentric A1 A7
  constraint perpendicular L0 L48
  constraint coincident L18 L48.end
  constraint coincident L19.start L48.start
  measures "d162" diameter of A4
extrude "돌출23" add sketch "스케치6" along normal blind 3 separate body contours L0 L1 L2 L3 L4 L5 L6 L7 L8 L9 L10 L11 L12 L13 L14 L15 L16 L17 L18 L19 L20 L21 L22 L23 L24 L25 L35 L39 L43 L47 L49 | L0 L4 L12 L14 L17 L18 L20 L48 | L0 L4 L17 L18 L19 L20 L21 L25 L48 | L0 L19 L21 L22 L25 L28 L30 L32 | L19 L22 L28 L32 L34 A4 | L3 L21 L25 L26 L28 L29 L30 L31 L32 L33 L34 L36 L37 L38 L40 L41 L42 L44 L45 L46 | L19 L22 L28 L34 L35 L36 | L28 L32 L33 L34 A4 | L3 L21 L24 L25 L26 L31 L46 L47 | L28 A4 | L28 A4 | L22 L28 L36 L38 A5 | L28 L36 L37 L38 A5 | L24 L26 L44 L46 A7 | L26 L44 L45 L46 A7 | L1 L2 L22 L23 L24 L26 L28 L29 L38 L39 L40 | L28 A5 | L28 A5 | L24 L26 L42 L43 L44 | L26 A7 | L26 A7 | L24 L26 L40 L42 A6 | L26 L40 L41 L42 A6 | L26 A6 | L26 A6 | A0 | A1 | A2 | A3 makes body 2
extrude "돌출24" add sketch "스케치6" against normal blind 6.5 contours L0 L4 L12 L14 L17 L18 L20 L48 | L0 L4 L17 L18 L19 L20 L21 L25 L48 bodies 2
extrude "돌출40" add sketch "스케치6" against normal blind 14 contours L0 L4 L12 L14 L17 L18 L20 L48 bodies 2
extrude "돌출28" add sketch "스케치6" against normal blind 5 contours L0 L19 L21 L22 L25 L28 L30 L32 | L19 L22 L28 L34 L35 L36 | L3 L21 L24 L25 L26 L31 L46 L47 | L1 L2 L22 L23 L24 L26 L28 L29 L38 L39 L40 | L24 L26 L42 L43 L44 bodies 2
extrude "돌출29" cut sketch "스케치6" against normal blind 1.5 from surface at 3 contours L28 A4 | L28 A4 | L28 A5 | L28 A5 | L26 A7 | L26 A7 | L26 A6 | L26 A6 | A0 | A1 | A2 | A3 bodies 2
extrude "돌출30" cut sketch "스케치6" along normal blind 3 contours A0 | A1 | A2 | A3 bodies 2